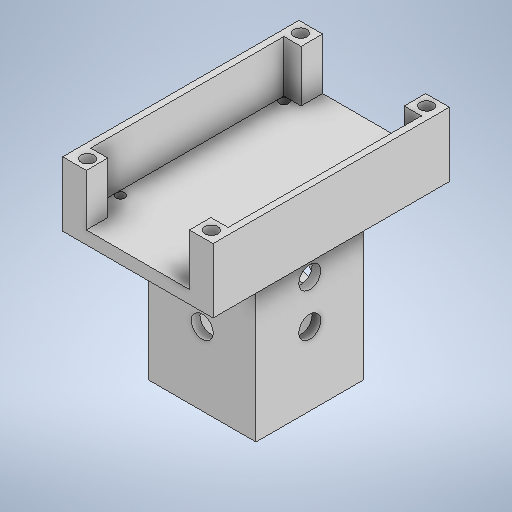
# Autodesk Inventor part: 零件3
Saved by Autodesk Inventor 2025.2 (Build 292293000, 293)
## iProperties
Created: 2025-07-02
Part Number: 零件3
Material: 一般
Document SubType Name: Modeling
Designer: 123
Density: 1 g/cm^3
Appearance: 預設
Author: 123
Autodesk Inventor part; units mm, degrees
ref_plane "YZ Plane" through (0, 0, 0) normal (1, 0, 0) x (0, 1, 0)
ref_plane "XZ Plane" through (0, 0, 0) normal (0, 1, 0) x (-1, 0, 0)
ref_plane "XY Plane" through (0, 0, 0) normal (0, 0, 1) x (1, 0, 0)
sketch "草圖1" plane through (0, 0, 0) normal (0, 1, 0) x (-1, 0, 0)
  line L0 (12.5, 12.5) -> (-12.5, 12.5)
  line L1 (-12.5, 12.5) -> (-12.5, -12.5)
  line L2 (-12.5, -12.5) -> (12.5, -12.5)
  line L3 (12.5, -12.5) -> (12.5, 12.5)
  line L4 (12.5, 12.5) -> (-12.5, -12.5) construction
  line L5 (-12.5, 12.5) -> (12.5, -12.5) construction
  point P0 (0, 0)
  dimension "d0" = 25
  dimension "d1" = 25
  constraints: 12 end point, 2 midpoint, 2 parallel, 1 horizontal, 1 perpendicular
  measures "d0" distance of L0.start L0.end
  measures "d1" distance of L2.end L0.start
extrude "擠出1" add sketch "草圖1" along normal blind 35
sketch "草圖2" plane through (0, 35, 0) normal (0, 1, 0) x (1, 0, 0)
  line L0 (-10.5, -10.5) -> (10.5, -10.5)
  line L1 (10.5, -10.5) -> (10.5, 10.5)
  line L2 (10.5, 10.5) -> (-10.5, 10.5)
  line L3 (-10.5, 10.5) -> (-10.5, -10.5)
  line L4 (-10.5, -10.5) -> (10.5, 10.5) construction
  line L5 (10.5, -10.5) -> (-10.5, 10.5) construction
  point P0 (0, 0)
  dimension "d4" = 21
  dimension "d5" = 21
  constraints: 12 end point, 2 midpoint, 2 parallel, 1 horizontal, 1 perpendicular
  measures "d4" distance of L2.end L0.start
  measures "d5" distance of L1.end L2.end
extrude "擠出2" cut sketch "草圖2" against normal through all
sketch "草圖3" plane through (-12.5, 0, 12.5) normal (0, 0, 1) x (1, 0, 0)
  line L0 (2, 35) -> (23, 35) projected
  line L1 (12.5, 35) -> (12.5, 0)
  circle A0 centre (12.5, 17) radius 2.55
  circle A1 centre (12.5, 27) radius 2.55
  line L2 (0, 0) -> (25, 0) projected
  point P0 (12.5, 0)
  dimension "d8" = 5.1
  dimension "d9" = 5.1
  dimension "d10" = 10
  dimension "d11" = 17
  constraints: 2 centre point, 2 end point, 2 midpoint, 2 point on line, 1 vertical
  measures "d8" diameter of A1
  measures "d9" diameter of A0
  measures "d10" distance of A0.centre A1.centre
  measures "d11" distance of point (12.5, 0) A0.centre
extrude "擠出3" cut sketch "草圖3" against normal through all
sketch "草圖4" plane through (0, 35, 0) normal (0, 1, 0) x (1, 0, 0)
  line L0 (-17.5, 27.5) -> (17.5, 27.5)
  line L1 (17.5, 27.5) -> (17.5, -27.5)
  line L2 (17.5, -27.5) -> (-17.5, -27.5)
  line L3 (-17.5, -27.5) -> (-17.5, 27.5)
  line L4 (-17.5, 27.5) -> (17.5, -27.5) construction
  line L5 (17.5, 27.5) -> (-17.5, -27.5) construction
  point P0 (0, 0)
  dimension "d14" = 55
  dimension "d15" = 35
  constraints: 12 end point, 2 midpoint, 2 parallel, 1 horizontal, 1 perpendicular
  measures "d14" distance of L2.end L0.start
  measures "d15" distance of L0.start L0.end
extrude "擠出4" add sketch "草圖4" along normal blind 15
sketch "草圖5" plane through (0, 50, 0) normal (0, 1, 0) x (1, 0, 0)
  line L0 (-16, -22.5) -> (16, -22.5)
  line L1 (16, -22.5) -> (16, 22.5)
  line L2 (16, 22.5) -> (-16, 22.5)
  line L3 (-16, 22.5) -> (-16, -22.5)
  line L4 (-16, -22.5) -> (16, 22.5) construction
  line L5 (16, -22.5) -> (-16, 22.5) construction
  point P0 (0, 0)
  dimension "d18" = 45
  dimension "d19" = 32
  constraints: 12 end point, 2 midpoint, 2 parallel, 1 horizontal, 1 perpendicular
  measures "d18" distance of L2.end L0.start
  measures "d19" distance of L1.end L2.end
extrude "擠出5" cut sketch "草圖5" against normal blind 12
sketch "草圖6" plane through (-17.5, 35, 27.5) normal (0, 0, 1) x (1, 0, 0)
  line L0 (0, 0) -> (0, 15) projected
  line L1 (0, 7.5) -> (35, 7.5)
  line L2 (35, 0) -> (35, 15) projected
  arc A0 (5.5, 7.5) -> (14.5, 7.5) centre (10, 7.5) ccw
  arc A1 (20.5, 7.5) -> (29.5, 7.5) centre (25, 7.5) ccw
  line L3 (35, 15) -> (0, 15) projected
  line L4 (17.5, 15) -> (17.5, 0)
  line L5 (0, 0) -> (35, 0) projected
  line L6 (5.5, 7.5) -> (14.5, 7.5)
  line L7 (14.5, 7.5) -> (14.5, 15)
  line L8 (14.5, 15) -> (5.5, 15)
  line L9 (5.5, 15) -> (5.5, 7.5)
  line L10 (20.5, 7.5) -> (29.5, 7.5)
  line L11 (29.5, 7.5) -> (29.5, 15)
  line L12 (29.5, 15) -> (20.5, 15)
  line L13 (20.5, 15) -> (20.5, 7.5)
  line L14 (14.5, 7.5) -> (20.5, 7.5)
  line L15 (1.5, 3) -> (33.5, 3) projected
  line L16 (5.5, 15) -> (29.5, 15)
  line L17 (29.5, 15) -> (29.5, 3)
  line L18 (29.5, 3) -> (5.5, 3)
  line L19 (5.5, 3) -> (5.5, 15)
  point P0 (17.5, -35)
  point P1 (20.5, 15)
  point P2 (29.5, 7.5)
  point P3 (28.5, 7.5)
  point P4 (29.5, 7.5)
  point P5 (5.5, 15)
  point P6 (14.5, 7.5)
  point P7 (13.5, 7.5)
  point P8 (25, 3)
  point P9 (10, 3)
  point P10 (25, 3)
  point P11 (29.5, 7.5)
  point P12 (5.5, 7.5)
  point P13 (5.5, 7.5)
  point P14 (29.5, 7.5)
  dimension "d22" = 9
  dimension "d23" = 9
  dimension "d24" = 15
  dimension "d25" = 7.5
  dimension "d52" = 24
  constraints: 30 end point, 7 point on line, 6 parallel, 4 midpoint, 4 point on circle, 3 horizontal, 3 perpendicular, 2 centre point, 2 tangent, 1 collinear
  measures "d22" diameter of A0
  measures "d23" diameter of A1
  measures "d24" distance of A1.centre A0.centre
  measures "d25" distance from line of L4 A1.centre
  measures "d52" distance of L17.end L18.end
extrude "擠出8" cut sketch "草圖6" against normal through all contours L9 L3 L7 L1 | L1 A0 | A0 L15 L19 | L15 A0 L1 L4 | L4 L1 A1 L15 | L7 L3 L4 L1 | L4 L3 L13 L1 | A1 L1 | A1 L17 L15 | L13 L3 L11 L1
sketch "草圖9" plane through (0, 50, 0) normal (0, 1, 0) x (1, 0, 0)
  circle A0 centre (-14.2115, -25) radius 1.5
  circle A1 centre (14.6091, -25) radius 1.5
  circle A2 centre (14.6091, 25.0995) radius 1.5
  circle A3 centre (-14.75, 25.0995) radius 1.5
  line L0 (-12, -27.5) -> (-12, -22.5) projected
  line L1 (-12, -25) -> (-17.5, -25)
  line L2 (-17.5, 27.5) -> (-17.5, -27.5) projected
  line L3 (17.5, -27.5) -> (17.5, 27.5) projected
  line L4 (17.5, -25) -> (-17.5, -25)
  line L5 (-17.5, 25.0938) -> (17.5, 25.0938)
  line L6 (14.6091, -25) -> (14.6091, 25.0995)
  line L7 (17.5, 27.5) -> (12, 27.5) projected
  line L8 (14.6091, 25.0995) -> (-14.75, 25.0995)
  line L9 (-14.75, 25.0995) -> (-14.75, -25)
  point P0 (0, 0)
  dimension "d34" = 3
  dimension "d35" = 3
  dimension "d36" = 3
  dimension "d37" = 3
  dimension "d38" = 0
  dimension "d39" = 0
  constraints: 12 end point, 5 point on line, 4 centre point, 3 perpendicular, 2 midpoint, 1 collinear, 1 horizontal, 1 parallel
  measures "d34" diameter of A0
  measures "d35" diameter of A1
  measures "d36" diameter of A3
  measures "d37" diameter of A2
  measures "d38" vertical distance of L9.end A0.centre
  measures "d39" distance from line of L4 L6.start
extrude "擠出9" cut sketch "草圖9" against normal blind 15 contours L1 L9 A0 | A0 L1 | L9 L1 A0 | L9 L5 A3 | A3 L5 L9 | L4 A1 | A1 L6 L4 | A3 L8 L9 L5 | L5 L9 L8 A3 | L8 L6 L5 | A2 L5 L6 L8 | L5 L6 A2 | A1 L4 L6 | L6 L5 A2
sketch "草圖11" plane through (12.5, 0, 12.5) normal (1, 0, 0) x (0, 0, -1)
  circle A0 centre (12.5, 27) radius 2.55
  circle A1 centre (12.5, 17) radius 2.55
  line L0 (0, 0) -> (25, 0) projected
  point P0 (12.5, 0)
  point P1 (12.5, 0)
  dimension "d46" = 5.1
  dimension "d47" = 5.1
  dimension "d48" = 17
  dimension "d49" = 10
  constraints: 2 centre point, 1 midpoint
  measures "d46" diameter of A0
  measures "d47" diameter of A1
  measures "d48" distance of point (12.5, 0) A1.centre
  measures "d49" distance of A1.centre A0.centre
extrude "擠出11" cut sketch "草圖11" against normal up to surface (25 mm away)
sketch "草圖12" plane through (0, 38, 0) normal (0, 1, 0) x (1, 0, 0)
  circle A0 centre (-14.95, 21.45) radius 1.05
  circle A1 centre (14.95, 21.45) radius 1.05
  line L0 (-16, 22.5) -> (-12, 22.5) projected
  line L1 (-16, -22.5) -> (-16, 22.5) projected
  line L2 (12, 22.5) -> (16, 22.5) projected
  line L3 (16, 22.5) -> (16, -22.5) projected
  circle A2 centre (-14.95, -16.55) radius 1.05
  circle A3 centre (14.95, -16.55) radius 1.05
  point P0 (0, 0)
  dimension "d53" = 2.1
  dimension "d54" = 2.1
  dimension "d55" = 2.1
  dimension "d56" = 2.1
  dimension "d57" = 38
  dimension "d58" = 38
  constraints: 6 tangent, 4 centre point
  measures "d53" diameter of A0
  measures "d54" diameter of A1
  measures "d55" diameter of A2
  measures "d56" diameter of A3
  measures "d57" distance of A2.centre A0.centre
  measures "d58" distance of A1.centre A3.centre
extrude "擠出12" cut sketch "草圖12" against normal up to surface (3 mm away) contours A0 | A2 | A1 | A3
